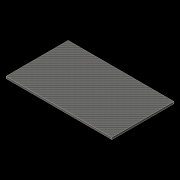
# Autodesk Inventor part: TheLid
Saved by Autodesk Inventor 2016 (Build 200138000, 138)
## iProperties
Created: 2017-02-08
Part Number: TheLid
Material: Generic
Document SubType Name: Modeling
Designer: Alexis Renderos
Density: 1 g/cm^3
Appearance: Diamond Plate
Author: Alexis Renderos
Autodesk Inventor part; units mm, degrees
ref_plane "YZ Plane" through (0, 0, 0) normal (1, 0, 0) x (0, 1, 0)
ref_plane "XZ Plane" through (0, 0, 0) normal (0, 1, 0) x (-1, 0, 0)
ref_plane "XY Plane" through (0, 0, 0) normal (0, 0, 1) x (1, 0, 0)
sketch "Sketch1" plane through (0, 0, 0) normal (0, 1, 0) x (-1, 0, 0)
  line L0 (0, -136.3015) -> (0, 136.3015) projected
  line L1 (-232.349, 0) -> (232.349, 0) projected
  line L2 (165.9636, 97.3582) -> (-165.9636, 97.3582)
  line L3 (-165.9636, 97.3582) -> (-165.9636, -97.3582)
  line L4 (-165.9636, -97.3582) -> (165.9636, -97.3582)
  line L5 (165.9636, -97.3582) -> (165.9636, 97.3582)
  point P0 (0, 0)
  dimension "d0" = 331.9272
  dimension "d1" = 194.7164
  constraints: 8 end point, 2 parallel, 1 horizontal, 1 perpendicular, 2 other
  measures "d0" distance of L4.end L3.end
  measures "d1" distance of L2.end L3.end
extrude "Extrusion1" add sketch "Sketch1" along normal mid plane 6.35
body "Solid1"
